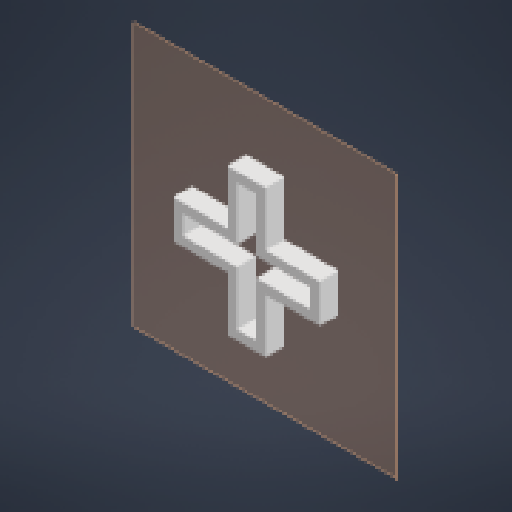
# Autodesk Inventor part: BetteKryds
Saved by Autodesk Inventor 2027 (Build 310192000, 192)
## iProperties
Created: 2026-03-31
Part Number: BetteKryds
Material: Generic
Document SubType Name: Modeling
Designer: Tueha
Density: 1 g/cm^3
Appearance: Default
Author: Tueha
Autodesk Inventor part; units mm, degrees
ref_plane "YZ Plane" through (0, 0, 0) normal (1, 0, 0) x (0, 1, 0)
ref_plane "XZ Plane" through (0, 0, 0) normal (0, 1, 0) x (-1, 0, 0)
ref_plane "XY Plane" through (0, 0, 0) normal (0, 0, 1) x (1, 0, 0)
ref_plane "Work Plane1" through (0, 0, 0) normal (0, 0, 1) x (1, 0, 0)
sketch "Sketch1" plane through (0, 0, 0) normal (0, 0, 1) x (1, 0, 0)
  line L0 (19.9, 3) -> (3, 3) construction
  line L1 (-19.9, 3) -> (19.9, 3) projected
  line L2 (19.9, 3) -> (19.9, -3) construction
  line L3 (3, 3) -> (3, 19.9) construction
  line L4 (-3, 19.9) -> (3, 19.9) construction
  line L5 (19.9, -3) -> (-19.9, -3) construction
  line L6 (3, -19.9) -> (3, -3) construction
  line L7 (-3, -19.9) -> (3, -19.9) construction
  line L8 (-3, -19.9) -> (-3, -3) projected
  line L9 (-19.9, -3) -> (-19.9, 3) construction
  line L10 (-3, 3) -> (-3, 19.9) construction
  line L11 (-3, 19.9) -> (3, 19.9) construction
  line L12 (-19.9, -3) -> (-19.9, 3) construction
  line L13 (3, -19.9) -> (3, -3) construction
  line L14 (19.9, 3) -> (19.9, -3)
  line L15 (19.9, -3) -> (3, -3)
  line L16 (3, -3) -> (3, -19.9)
  line L17 (3, -19.9) -> (-3, -19.9)
  line L18 (-3, -3) -> (-19.9, -3)
  line L19 (-19.9, -3) -> (-19.9, 3)
  line L20 (-3, 3) -> (-19.9, 3)
  line L21 (-3, 3) -> (-3, 19.9)
  line L22 (-3, 19.9) -> (3, 19.9)
  line L23 (3, 19.9) -> (3, 3)
  line L24 (3, 3) -> (19.9, 3)
  line L25 (-3, -19.9) -> (-3, -3)
  line L26 (6, -22.9) -> (6, -6)
  line L27 (6, -6) -> (22.9, -6)
  line L28 (22.9, -6) -> (22.9, 6)
  line L29 (22.9, 6) -> (6, 6)
  line L30 (6, 6) -> (6, 22.9)
  line L31 (6, 22.9) -> (-6, 22.9)
  line L32 (-6, 22.9) -> (-6, 6)
  line L33 (-6, 6) -> (-22.9, 6)
  line L34 (-22.9, 6) -> (-22.9, -6)
  line L35 (-22.9, -6) -> (-6, -6)
  line L36 (-6, -6) -> (-6, -22.9)
  line L37 (-6, -22.9) -> (6, -22.9)
  point P0 (0, 0)
  dimension "d0" = 3
  constraints: 48 end point, 9 perpendicular, 6 collinear, 11 other
  measures "d0" distance between parallel lines of L16 L26
extrude "Extrusion1" add sketch "Sketch1" along normal blind 6
body "Solid1"
